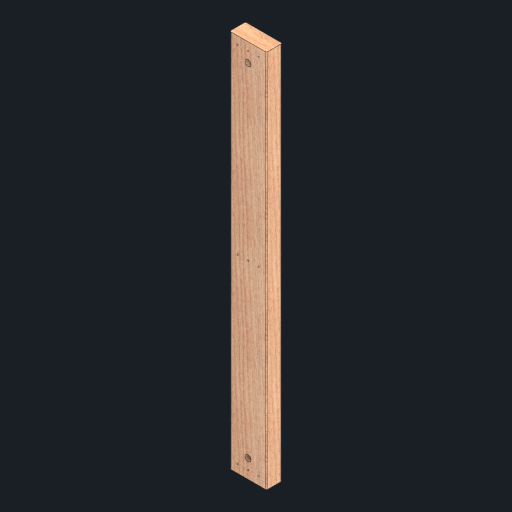
# Autodesk Inventor part: Horizontal Beam 3ft
Saved by Autodesk Inventor 2024.2 (Build 282272000, 272)
## iProperties
Created: 2025-06-28
Part Number: Horizontal Beam 3ft
Material: Wood (Birch)
Document SubType Name: Modeling
Designer: Bryan
Density: 0.55 g/cm^3
Appearance: Birch - Natural Polished
Mass: 1685.83 g
Surface Area: 2409.96 cm^2
Volume: 3065.15 cm^3
Author: Bryan
Autodesk Inventor part; units mm, degrees
ref_plane "YZ Plane" through (0, 0, 0) normal (1, 0, 0) x (0, 1, 0)
ref_plane "XZ Plane" through (0, 0, 0) normal (0, 1, 0) x (-1, 0, 0)
ref_plane "XY Plane" through (0, 0, 0) normal (0, 0, 1) x (1, 0, 0)
sketch "Sketch1" plane through (0, 0, 0) normal (0, 1, 0) x (-1, 0, 0)
  line L0 (3.175, 0) -> (85.725, 0)
  line L1 (88.9, -3.175) -> (88.9, -34.925)
  line L2 (85.725, -38.1) -> (3.175, -38.1)
  line L3 (0, -34.925) -> (0, -3.175)
  arc A0 (88.9, -3.175) -> (85.725, 0) centre (85.725, -3.175) ccw
  arc A1 (85.725, -38.1) -> (88.9, -34.925) centre (85.725, -34.925) ccw
  arc A2 (0, -34.925) -> (3.175, -38.1) centre (3.175, -34.925) ccw
  arc A3 (3.175, 0) -> (0, -3.175) centre (3.175, -3.175) ccw
  point P0 (0, 0)
  point P1 (88.9, -38.1)
  point P2 (88.9, 0)
  point P3 (0, -38.1)
  dimension "d0" = 88.9
  dimension "d1" = 38.1
  dimension "d2" = 3.175
  constraints: 8 end point, 8 point on circle, 8 point on line, 8 tangent, 4 centre point, 3 equal radius, 2 parallel, 1 horizontal, 1 perpendicular
  measures "d0" distance of point (88.9, -38.1) point (0, -38.1)
  measures "d1" distance of point (88.9, 0) point (88.9, -38.1)
  measures "d2" radius of A0
extrude "Extrusion1" add sketch "Sketch1" along normal blind 914.4
sketch "Sketch2" plane through (-85.725, 0, 0) normal (0, 0, 1) x (1, 0, 0)
  line L0 (0, 0) -> (82.55, 0) construction
  line L1 (82.55, 0) -> (82.55, 914.4) construction
  line L2 (0, 914.4) -> (82.55, 914.4) construction
  line L3 (0, 0) -> (0, 914.4) construction
  line L4 (-3.175, 0) -> (-3.175, 914.4) construction
  line L5 (85.725, 0) -> (85.725, 914.4) construction
  circle A0 centre (41.275, 44.45) radius 7.3025
  line L6 (41.275, 0) -> (41.275, 44.45) construction
  line L7 (41.275, 44.45) -> (-3.175, 44.45) construction
  line L8 (-3.175, 0) -> (-3.175, 914.4) construction
  line L9 (-3.175, 457.2) -> (85.725, 457.2) construction
  circle A1 centre (41.275, 869.95) radius 7.3025
  dimension "d5" = 14.605
  constraints: 6 end point, 3 midpoint, 2 centre point, 1 horizontal, 1 perpendicular, 1 point on line, 1 symmetric about line, 1 vertical, 1 vertical alignment, 1 other
  measures "d5" diameter of A0
extrude "Extrusion2" cut sketch "Sketch2" against normal through all
sketch "Sketch3" plane through (-85.725, 0, -38.1) normal (0, 0, 1) x (1, 0, 0)
  circle A0 centre (41.275, 44.45) radius 7.3025 projected
  circle A1 centre (41.275, 44.45) radius 12.7
  line L0 (0, 0) -> (0, 914.4) construction
  line L1 (0, 457.2) -> (82.55, 457.2) construction
  line L2 (82.55, 0) -> (82.55, 914.4) construction
  circle A2 centre (41.275, 869.95) radius 12.7
  point P0 (85.725, 0)
  dimension "d8" = 25.4
  constraints: 2 centre point, 2 end point, 2 midpoint, 1 coincident, 1 symmetric about line, 1 other
  measures "d8" diameter of A1
extrude "Extrusion3" cut sketch "Sketch3" along normal blind 12.7 contours A0 | A1 | A2
sketch "Sketch4" plane through (-85.725, 0, 0) normal (0, 0, 1) x (1, 0, 0)
  line L0 (85.725, 0) -> (-3.175, 0) construction
  line L1 (-3.175, 0) -> (-3.175, 38.1) construction
  line L2 (-3.175, 38.1) -> (85.725, 38.1) construction
  line L3 (85.725, 38.1) -> (85.725, 0) construction
  circle A0 centre (66.675, 19.05) radius 19.05 construction
  line L4 (0, 0) -> (82.55, 0) projected
  circle A1 centre (15.875, 19.05) radius 19.05 construction
  circle A2 centre (66.675, 19.05) radius 1.5875
  circle A3 centre (15.875, 19.05) radius 1.5875
  circle A4 centre (41.275, 19.05) radius 1.5875
  line L5 (0, 0) -> (0, 914.4) projected
  line L6 (0, 457.2) -> (82.55, 457.2) construction
  line L7 (82.55, 0) -> (82.55, 914.4) projected
  line L8 (85.725, 438.15) -> (-3.175, 438.15) construction
  line L9 (-3.175, 438.15) -> (-3.175, 476.25) construction
  line L10 (-3.175, 476.25) -> (85.725, 476.25) construction
  line L11 (85.725, 476.25) -> (85.725, 438.15) construction
  circle A5 centre (66.675, 457.2) radius 19.05 construction
  circle A6 centre (15.875, 457.2) radius 19.05 construction
  circle A7 centre (66.675, 457.2) radius 1.5875
  circle A8 centre (15.875, 457.2) radius 1.5875
  circle A9 centre (41.275, 457.2) radius 1.5875
  circle A10 centre (66.675, 895.35) radius 1.5875
  circle A11 centre (15.875, 895.35) radius 1.5875
  circle A12 centre (41.275, 895.35) radius 1.5875
  point P0 (41.275, 0)
  point P1 (41.275, 438.15)
  point P2 (41.275, 457.2)
  dimension "d11" = 88.9
  dimension "d12" = 38.1
  dimension "d13" = 3.175
  dimension "d14" = 88.9
  dimension "d15" = 38.1
  dimension "d16" = 3.175
  constraints: 18 end point, 13 centre point, 12 tangent, 5 coincident, 5 midpoint, 4 equal radius, 4 parallel, 3 symmetric about line, 2 horizontal, 2 horizontal alignment, 2 perpendicular, 2 vertical alignment, 3 other
  measures "d11" distance of L1.end L2.end
  measures "d12" distance of L0.end L1.end
  measures "d13" diameter of A2
  measures "d14" distance of L9.end L10.end
  measures "d15" distance of L8.end L9.end
  measures "d16" diameter of A7
extrude "Extrusion4" cut sketch "Sketch4" against normal through all
body "Solid1"
